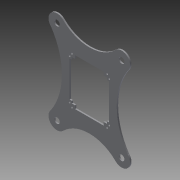
# Autodesk Inventor part: atas4
Saved by Autodesk Inventor 2015 (Build 190159000, 159)
## iProperties
Created: 2015-01-14
Part Number: atas4
Material: Generic
Document SubType Name: Modeling
Designer: Rafi Kurnia Putra
Density: 1 g/cm^3
Appearance: Default
Author: Rafi Kurnia Putra
Autodesk Inventor part; units mm, degrees
ref_plane "YZ Plane" through (0, 0, 0) normal (1, 0, 0) x (0, 1, 0)
ref_plane "XZ Plane" through (0, 0, 0) normal (0, 1, 0) x (-1, 0, 0)
ref_plane "XY Plane" through (0, 0, 0) normal (0, 0, 1) x (1, 0, 0)
sketch "Sketch1" plane through (0, 0, 0) normal (0, 1, 0) x (-1, 0, 0)
  circle A0 centre (-28.625, 29.0323) radius 1.5
  circle A1 centre (-25.375, 33.6573) radius 1.5
  arc A2 (-37.9702, 69.5664) -> (0, 53.8386) centre (0, 107.5366) ccw
  arc A3 (-39.6019, 0) -> (-55.3297, 52.2069) centre (-134.1138, 0) ccw
  circle A4 centre (-46.65, 60.8866) radius 4.05
  arc A5 (-37.9702, 69.5664) -> (-55.3297, 52.2069) centre (-46.65, 60.8866) ccw
  arc A6 (-55.3297, -52.2069) -> (-39.6019, 0) centre (-134.1138, 0) ccw
  circle A7 centre (-28.625, -29.0323) radius 1.5
  circle A8 centre (-25.375, -33.6573) radius 1.5
  circle A9 centre (-46.65, -60.8866) radius 4.05
  arc A10 (-55.3297, -52.2069) -> (-37.9702, -69.5664) centre (-46.65, -60.8866) ccw
  arc A11 (0, -53.8386) -> (-37.9702, -69.5664) centre (0, -107.5366) ccw
  arc A12 (39.6019, 0) -> (55.3297, -52.2069) centre (134.1138, 0) ccw
  circle A13 centre (28.625, -29.0323) radius 1.5
  circle A14 centre (25.375, -33.6573) radius 1.5
  arc A15 (37.9702, -69.5664) -> (0, -53.8386) centre (0, -107.5366) ccw
  circle A16 centre (46.65, -60.8866) radius 4.05
  arc A17 (37.9702, -69.5664) -> (55.3297, -52.2069) centre (46.65, -60.8866) ccw
  circle A18 centre (28.625, 29.0323) radius 1.5
  circle A19 centre (25.375, 33.6573) radius 1.5
  arc A20 (0, 53.8386) -> (37.9702, 69.5664) centre (0, 107.5366) ccw
  arc A21 (55.3297, 52.2069) -> (39.6019, 0) centre (134.1138, 0) ccw
  circle A22 centre (46.65, 60.8866) radius 4.05
  arc A23 (55.3297, 52.2069) -> (37.9702, 69.5664) centre (46.65, 60.8866) ccw
  arc A24 (55.3297, 52.2069) -> (37.9702, 69.5664) centre (46.65, 60.8866) ccw
  arc A25 (-37.9702, 69.5664) -> (-55.3297, 52.2069) centre (-46.65, 60.8866) ccw
  arc A26 (-55.3297, -52.2069) -> (-37.9702, -69.5664) centre (-46.65, -60.8866) ccw
  circle A27 centre (-46.65, -60.8866) radius 4.05
  circle A28 centre (46.65, -60.8866) radius 4.05
  circle A29 centre (46.65, 60.8866) radius 4.05
  circle A30 centre (-46.65, 60.8866) radius 4.05
  circle A31 centre (-25.375, -33.6573) radius 1.5
  circle A32 centre (-28.625, -29.0323) radius 1.5
  circle A33 centre (25.375, -33.6573) radius 1.5
  circle A34 centre (28.625, -29.0323) radius 1.5
  circle A35 centre (28.625, 29.0323) radius 1.5
  circle A36 centre (25.375, 33.6573) radius 1.5
  circle A37 centre (-28.625, 29.0323) radius 1.5
  circle A38 centre (-25.375, 33.6573) radius 1.5
  arc A39 (-37.9702, 69.5664) -> (37.9702, 69.5664) centre (0, 107.5366) ccw
  arc A40 (55.3297, 52.2069) -> (55.3297, -52.2069) centre (134.1138, 0) ccw
  arc A41 (-55.3297, -52.2069) -> (-55.3297, 52.2069) centre (-134.1138, 0) ccw
  arc A42 (37.9702, -69.5664) -> (-37.9702, -69.5664) centre (0, -107.5366) ccw
  line L0 (28.625, -25.7823) -> (25.375, -25.7823)
  line L1 (25.375, 25.7823) -> (28.625, 25.7823)
  line L2 (28.625, 25.7823) -> (28.625, -25.7823)
  line L3 (-28.625, -25.7823) -> (-25.375, -25.7823)
  line L4 (-25.375, 25.7823) -> (-28.625, 25.7823)
  line L5 (-28.625, 25.7823) -> (-28.625, -25.7823)
  line L6 (20.75, -33.6573) -> (-20.75, -33.6573)
  line L7 (-20.75, -33.6573) -> (-20.75, -29.0323)
  line L8 (20.75, -29.0323) -> (20.75, -33.6573)
  line L9 (20.75, 33.6573) -> (-20.75, 33.6573)
  line L10 (-20.75, 33.6573) -> (-20.75, 29.0323)
  line L11 (20.75, 29.0323) -> (20.75, 33.6573)
  line L12 (25.375, 29.0323) -> (25.375, 25.7823)
  line L13 (25.375, -25.7823) -> (25.375, -29.0323)
  line L14 (25.375, -29.0323) -> (20.75, -29.0323)
  line L15 (-20.75, -29.0323) -> (-25.375, -29.0323)
  line L16 (-25.375, -29.0323) -> (-25.375, -25.7823)
  line L17 (-25.375, 25.7823) -> (-25.375, 29.0323)
  line L18 (-25.375, 29.0323) -> (-20.75, 29.0323)
  line L19 (20.75, 29.0323) -> (25.375, 29.0323)
  point P0 (-25.25, 18.3592)
  point P1 (-4.2075, 54.5249)
  point P2 (-4.2075, -54.5249)
  point P3 (25.25, 18.3592)
  point P4 (4.2075, -54.5249)
  point P5 (4.2075, 54.5249)
  dimension "d0" = 3.25
  dimension "d1" = 3.25
  dimension "d2" = 4.625
  dimension "d3" = 4.625
  constraints: 50 point on circle, 43 centre point, 40 end point, 18 coincident, 18 concentric, 10 parallel, 5 perpendicular, 4 horizontal, 2 vertical, 4 other
  measures "d0" distance of L0.start A13.centre
  measures "d1" distance of L1.end A18.centre
  measures "d2" distance of L6.start A33.centre
  measures "d3" distance from line of A8.centre L7
extrude "Extrusion1" add sketch "Sketch1" along normal blind 2
body "Solid1"
